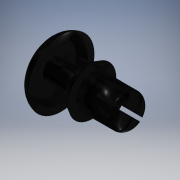
# Autodesk Inventor part: 11-6001
Saved by Autodesk Inventor 2017.1 (Build 211199000, 199)
## iProperties
Category: Quick Connect Service Pack
Company: Autodesk Inc.
Created: 2014-11-30
Part Number: 11-6001
Material: Polystyrene, High Impact
Document SubType Name: Modeling
Designer: Matrix
Density: 1.022 g/cm^3
Appearance: Black
Catalog Web Link: http://matrixrobotics.com/
Vendor: Matrix
Author: Autodesk Inc.
Autodesk Inventor part; units mm, degrees
ref_plane "YZ Plane" through (0, 0, 0) normal (1, 0, 0) x (0, 1, 0)
ref_plane "XZ Plane" through (0, 0, 0) normal (0, 1, 0) x (-1, 0, 0)
ref_plane "XY Plane" through (0, 0, 0) normal (0, 0, 1) x (1, 0, 0)
sketch "Sketch1" plane through (0, 0, 0) normal (0, 1, 0) x (-1, 0, 0)
  arc A0 (2.5786, 4.3289) -> (0, 4.6354) centre (0, -6.3646) ccw
  arc A1 (4, 2.8354) -> (2.5786, 4.3289) centre (2.1332, 2.4819) ccw
  line L0 (4, 2.8354) -> (3.2, 2.8354)
  line L1 (3.2, 2.8354) -> (2.8, 3.8354)
  line L2 (2.8, 3.8354) -> (1.225, 3.8354)
  line L3 (1.225, 3.8354) -> (1.225, -0.9)
  line L4 (1.225, -0.9) -> (1.275, -0.9)
  line L5 (1.275, -0.9) -> (1.275, 0)
  line L6 (1.275, 0) -> (2.3804, 0)
  line L7 (2.3804, 0) -> (2.9, -0.9)
  line L8 (2.9, -0.9) -> (1.99, -0.9)
  line L9 (1.275, -1.5) -> (1.225, -1.5)
  arc A2 (2.5786, 4.3289) -> (0, 4.6354) centre (0, -6.3646) ccw
  arc A3 (4, 2.8354) -> (2.5786, 4.3289) centre (2.1332, 2.4819) ccw
  line L10 (4, 2.8354) -> (3.2, 2.8354)
  line L11 (3.2, 2.8354) -> (2.8, 3.8354)
  line L12 (2.8, 3.8354) -> (1.225, 3.8354)
  line L13 (1.225, 3.8354) -> (1.225, -0.9)
  line L14 (1.225, -0.9) -> (1.275, -0.9)
  line L15 (1.275, -0.9) -> (1.275, 0)
  line L16 (1.275, 0) -> (2.3804, 0)
  line L17 (2.3804, 0) -> (2.9, -0.9)
  line L18 (2.9, -0.9) -> (2, -0.9)
  line L19 (1.275, -1.5) -> (1.225, -1.5)
  line L20 (1.99, -4.9) -> (1.99, -0.9)
  spline S0 degree 3 poles (1.99, -4.9) (1.99, -5.0231) (1.9611, -5.1679) (1.8666, -5.3956) (1.7841, -5.5186) (1.6089, -5.6933) (1.4849, -5.7757) (1.2538, -5.871) (1.1056, -5.9) (0.9798, -5.9) knots -0.250479 -0.250479 -0.250479 -0.250479 -0.213555 -0.213555 -0.176537 -0.176537 -0.139311 -0.139311 -0.101565 -0.101565 -0.101565 -0.101565
  line L21 (0, -5.9) -> (1, -5.9)
  line L22 (0, 4.6354) -> (0, -5.9)
  point P0 (0, 0)
  point P1 (0, 0)
  constraints: 46 end point, 8 point on circle, 4 centre point, 1 point on line, 1 vertical, 2 other
revolve "Revolution1" add sketch "Sketch1" angle 360 about axis through (0, 0, 4.6354) along (0, 0, -1)
sketch "Sketch2" plane through (0, 0, -5.9) normal (0, 0, -1) x (-1, 0, 0)
  line L0 (0.8343, -0.5514) -> (0.2829, 0)
  line L1 (0.2829, 0) -> (0.8343, 0.5514)
  arc A0 (0.8343, -0.5514) -> (0.8343, 0.5514) centre (0, 0) ccw
  line L2 (-0.5514, -0.8343) -> (0, -0.2829)
  line L3 (0, -0.2829) -> (1.2657, -1.5486)
  arc A1 (-0.5514, -0.8343) -> (0.5514, -0.8343) centre (0, 0) ccw
  line L4 (-0.2829, 0) -> (-1.5486, -1.2657)
  arc A2 (-0.8343, 0.5514) -> (-0.8343, -0.5514) centre (0, 0) ccw
  line L5 (-0.8343, 0.5514) -> (-0.2829, 0)
  line L6 (0, 0.2829) -> (-1.2657, 1.5485)
  arc A3 (0.5514, 0.8343) -> (-0.5514, 0.8343) centre (0, 0) ccw
  line L7 (1.2657, 1.5486) -> (0, 0.2829)
  circle A4 centre (0, 0) radius 2.9
  line L8 (-1.2657, -1.5485) -> (-0.5514, -0.8343)
  line L9 (-1.5485, 1.2657) -> (-0.8343, 0.5514)
  line L10 (1.5485, -1.2656) -> (0.8343, -0.5514)
  line L11 (0.8343, 0.5514) -> (1.5485, 1.2657)
  arc A5 (1.2656, -1.5485) -> (1.5485, -1.2656) centre (0, 0) ccw
  arc A6 (-1.5485, -1.2656) -> (-1.2656, -1.5485) centre (0, 0) ccw
  arc A7 (1.5485, 1.2657) -> (1.2657, 1.5485) centre (0, 0) ccw
  arc A8 (-1.2656, 1.5485) -> (-1.5485, 1.2656) centre (0, 0) ccw
  point P0 (0, 0)
  constraints: 25 end point, 16 point on circle, 10 point on line, 9 centre point, 1 coincident
extrude "Extrusion1" cut sketch "Sketch2" against normal blind 3 contours L10 A5 L3 L2 L8 A6 L4 L5 L9 A8 L6 L7 A7 L11 L1 L0
body "Solid1"
